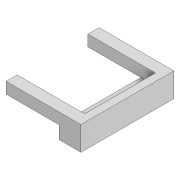
# Autodesk Inventor part: CentrationTool
Saved by Autodesk Inventor 2021 (Build 250183000, 183)
## iProperties
Created: 2021-08-07
Part Number: CentrationTool
Material: Generisch
Document SubType Name: Modeling
Designer: Rama
Density: 1 g/cm^3
Appearance: Vorgabe
Author: Rama
Autodesk Inventor part; units mm, degrees
ref_plane "YZ Plane" through (0, 0, 0) normal (1, 0, 0) x (0, 1, 0)
ref_plane "XZ Plane" through (0, 0, 0) normal (0, 1, 0) x (-1, 0, 0)
ref_plane "XY Plane" through (0, 0, 0) normal (0, 0, 1) x (1, 0, 0)
sketch "Skizze1" plane through (0, 0, 0) normal (0, 1, 0) x (-1, 0, 0)
  line L0 (9.105, 12) -> (-9.105, 12)
  line L1 (-9.105, 12) -> (-9.105, -12)
  line L2 (-9.105, -12) -> (9.105, -12)
  line L3 (9.105, -12) -> (9.105, 12)
  line L4 (9.105, 12) -> (-9.105, -12) construction
  line L5 (-9.105, 12) -> (9.105, -12) construction
  point P0 (0, 0)
  dimension "d0" = 18.21
  dimension "d1" = 24
  constraints: 12 end point, 2 midpoint, 2 parallel, 1 horizontal, 1 perpendicular
  measures "d0" distance of L2.end L1.end
  measures "d1" distance of L1.end L0.end
extrude "Extrusion1" add sketch "Skizze1" along normal blind 3.5
sketch "Skizze2" plane through (0, 3.5, 0) normal (0, 1, 0) x (1, 0, 0)
  line L0 (9.105, -12) -> (9.105, 12) projected
  line L1 (9.105, 12) -> (-9.105, 12) projected
  line L2 (9.105, -12) -> (5.195, -12)
  line L3 (5.195, -12) -> (5.195, 12)
  line L4 (5.195, 12) -> (9.105, 12)
  line L5 (9.105, 12) -> (9.105, -12)
  line L6 (9.105, -12) -> (9.105, 12) projected
  line L7 (9.105, 12) -> (-9.105, 12) projected
  line L8 (-9.105, 12) -> (-9.105, -12) projected
  line L9 (-9.105, -12) -> (9.105, -12) projected
  point P0 (0, 0)
  dimension "d4" = 3.91
  constraints: 8 end point, 2 parallel, 1 horizontal, 1 perpendicular, 1 point on line
  measures "d4" distance of L3.end L4.end
extrude "Extrusion2" cut sketch "Skizze2" against normal through all contours L9 L8 L1 L3
sketch "Skizze3" plane through (0, 3.5, 0) normal (0, 1, 0) x (1, 0, 0)
  line L0 (13.39, -9.55) -> (-3, -9.55)
  line L1 (-3, -9.55) -> (-3, 9.55)
  line L2 (-3, 9.55) -> (13.39, 9.55)
  line L3 (13.39, 9.55) -> (13.39, -9.55)
  line L4 (5.195, 12) -> (5.195, -12) projected
  line L5 (13.39, -9.55) -> (-3, 9.55) construction
  line L6 (-3, -9.55) -> (13.39, 9.55) construction
  line L7 (9.105, -12) -> (9.105, 12) projected
  line L8 (9.105, -9.55) -> (-9.105, -9.55)
  line L9 (-9.105, -9.55) -> (-9.105, -12.55)
  line L10 (-9.105, -12.55) -> (9.105, -12.55)
  line L11 (9.105, -12.55) -> (9.105, -9.55)
  line L12 (9.105, 9.55) -> (-9.105, 9.55)
  line L13 (-9.105, 9.55) -> (-9.105, 12.55)
  line L14 (-9.105, 12.55) -> (9.105, 12.55)
  line L15 (9.105, 12.55) -> (9.105, 9.55)
  point P0 (0, 0)
  point P1 (5.195, 0)
  dimension "d7" = 19.1
  dimension "d8" = 18.21
  dimension "d9" = 3
  dimension "d10" = 18.21
  dimension "d11" = 3
  constraints: 28 end point, 6 parallel, 4 point on line, 3 horizontal, 3 midpoint, 3 perpendicular
  measures "d7" distance of L0.end L1.end
  measures "d8" distance of L10.end L9.end
  measures "d9" distance of L9.end L8.end
  measures "d10" distance of L13.end L14.end
  measures "d11" distance of L12.end L13.end
extrude "Extrusion3" add sketch "Skizze3" along normal blind 3 contours L7 L11 L10 L9 L8 L0 | L2 L12 L13 L14 L15 L7
sketch "Skizze4" plane through (0, 3.5, 0) normal (0, -1, 0) x (1, 0, 0)
  line L0 (5.195, 12) -> (9.105, 12) projected
  line L1 (9.105, 12.55) -> (9.105, 12) projected
  line L2 (-9.105, 12.55) -> (9.105, 12.55) projected
  line L3 (-9.105, 9.55) -> (-9.105, 12.55) projected
  line L4 (5.195, 9.55) -> (-9.105, 9.55) projected
  line L5 (5.195, 9.55) -> (5.195, 12) projected
  line L6 (5.195, -12) -> (5.195, -9.55) projected
  line L7 (-9.105, -9.55) -> (5.195, -9.55) projected
  line L8 (-9.105, -12.55) -> (-9.105, -9.55) projected
  line L9 (9.105, -12.55) -> (-9.105, -12.55) projected
  line L10 (9.105, -12) -> (9.105, -12.55) projected
  line L11 (9.105, -12) -> (5.195, -12) projected
  line L12 (9.105, 12.55) -> (9.105, 12) projected
  line L13 (9.105, 12.55) -> (5.195, 12.55)
  line L14 (5.195, 12.55) -> (5.195, 9.55)
  line L15 (5.195, 9.55) -> (9.105, 9.55)
  line L16 (9.105, 9.55) -> (9.105, 12.55)
  line L17 (9.105, -12.55) -> (-9.105, -12.55) projected
  line L18 (5.195, -9.55) -> (5.195, 9.55) projected
  line L19 (9.105, -12.55) -> (5.195, -12.55)
  line L20 (5.195, -12.55) -> (5.195, -9.55)
  line L21 (5.195, -9.55) -> (9.105, -9.55)
  line L22 (9.105, -9.55) -> (9.105, -12.55)
  point P0 (0, 0)
  constraints: 16 end point, 4 parallel, 2 horizontal, 2 perpendicular
extrude "Extrusion4" add sketch "Skizze4" along normal up to surface (3.5 mm away) contours L14 L2 L1 L0 | L0 L16 L15 L5 | L21 L22 L11 L6 | L11 L10 L9 L20
sketch "Skizze5" plane through (9.105, 0, 12.55) normal (1, 0, 0) x (0, 0, -1)
  line L0 (0, 3.5) -> (0, 0) projected
  line L1 (0, 0) -> (25.1, 0)
  line L2 (25.1, 0) -> (25.1, 6.5)
  line L3 (25.1, 6.5) -> (0, 6.5)
  line L4 (0, 6.5) -> (0, 0)
  point P0 (12.55, 0)
  constraints: 8 end point, 2 parallel, 1 horizontal, 1 perpendicular
extrude "Extrusion5" add sketch "Skizze5" along normal blind 2
